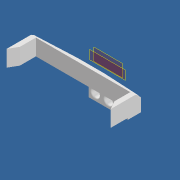
# Autodesk Inventor part: Hand
Saved by Autodesk Inventor 2020 (Build 240168000, 168)
## iProperties
Created: 2019-12-15
Part Number: Hand
Material: Generic
Document SubType Name: Modeling
Designer: Jack
Density: 1 g/cm^3
Appearance: Default
Author: Jack
Autodesk Inventor part; units mm, degrees
ref_plane "YZ Plane" through (0, 0, 0) normal (1, 0, 0) x (0, 1, 0)
ref_plane "XZ Plane" through (0, 0, 0) normal (0, 1, 0) x (-1, 0, 0)
ref_plane "XY Plane" through (0, 0, 0) normal (0, 0, 1) x (1, 0, 0)
sketch "Sketch1" plane through (0, 0, 0) normal (0, 0, 1) x (1, 0, 0)
  line L0 (32, -5) -> (-32, -5)
  line L1 (-32, -5) -> (-32, 5)
  line L2 (-32, 5) -> (32, 5)
  line L3 (32, 5) -> (32, -5)
  line L4 (32, -5) -> (-32, 5) construction
  line L5 (-32, -5) -> (32, 5) construction
  point P0 (0, 0)
  dimension "d1" = 64
  dimension "d2" = 10
  constraints: 12 end point, 2 midpoint, 2 parallel, 1 horizontal, 1 perpendicular
  measures "d1" distance of L1.end L2.end
  measures "d2" distance of L0.end L1.end
extrude "Extrusion1" add sketch "Sketch1" against normal blind 5
chamfer "Chamfer1" distance 24 distance2 3 1 edges at (32, 0, -5) measured on face at (31.5, 0, -5)
chamfer "Chamfer2" distance 24 distance2 3 1 edges at (-32, 0, -5) measured on face at (-31.5, 0, -5)
chamfer "Chamfer3" distance 3 distance2 5 1 edges at (0, 5, -5) measured on face at (0, 4.5, -5)
sketch "Sketch2" plane through (0, 0, 0) normal (0, 0, 1) x (1, 0, 0)
  line L0 (-32, 5) -> (-29, 5)
  line L1 (-29, 5) -> (-29, -5)
  line L2 (-29, -5) -> (-32, -5)
  line L3 (-32, -5) -> (-32, 5)
  line L4 (32, 5) -> (-32, 5) projected
  line L5 (-32, 5) -> (-32, -5) projected
  point P0 (0, 0)
  dimension "d14" = 3
  dimension "d15" = 10
  constraints: 8 end point, 2 collinear, 2 parallel, 1 horizontal, 1 perpendicular
  measures "d14" distance of L1.end L2.end
  measures "d15" distance of L0.end L1.end
extrude "Extrusion2" add sketch "Sketch2" along normal blind 15
chamfer "Chamfer4" distance 3 angle 60 1 edges at (-29, 0, 15) measured on face at (-29.5, 0, 15)
ref_plane "Work Plane1" through (0, 0, -15) normal (0, 0, -1) x (-1, 0, 0)
mirror "Mirror3" about plane through (0, 0, 0) normal (1, 0, 0)
ref_plane "Work Plane8" through (0, 0, -15.5) normal (0, 0, -1) x (-1, 0, 0)
sketch "Sketch19" plane through (0, 0, -15.5) normal (0, 0, -1) x (-1, 0, 0)
  line L0 (-12, -26) -> (12, -26)
  line L1 (12, -26) -> (12, -18)
  line L2 (12, -18) -> (-12, -18)
  line L3 (-12, -18) -> (-12, -26)
  line L4 (-12, -26) -> (12, -18) construction
  line L5 (12, -26) -> (-12, -18) construction
  line L6 (0, -32.2) -> (0, 11.2) projected
  line L7 (8, -5) -> (32, -5) projected
  point P0 (0, 0)
  point P1 (0, -22)
  point P2 (0, -22)
  dimension "d95" = 24
  dimension "d96" = 8
  dimension "d97" = 13
  constraints: 12 end point, 3 midpoint, 2 parallel, 1 horizontal, 1 perpendicular, 1 point on line
  measures "d95" distance of L2.end L1.end
  measures "d96" distance of L1.end L0.end
  measures "d97" distance between parallel lines of L7 L2
extrude "Extrusion9" add sketch "Sketch19" along normal blind 8
sketch "Sketch20" plane through (0, 0, -23.5) normal (0, 0, -1) x (-1, 0, 0)
  circle A0 centre (-8, -22) radius 2.4
  circle A1 centre (0, -22) radius 2.4
  circle A2 centre (8, -22) radius 2.4
  line L0 (0, -32.2) -> (0, 11.2) projected
  line L1 (12, -18) -> (-12, -18) projected
  point P0 (0, 0)
  dimension "d100" = 4.8
  dimension "d101" = 4.8
  dimension "d102" = 4.8
  dimension "d103" = 8
  dimension "d104" = 8
  dimension "d105" = 4
  constraints: 3 centre point, 2 horizontal alignment, 1 point on line
  measures "d100" diameter of A0
  measures "d101" diameter of A1
  measures "d102" diameter of A2
  measures "d103" distance of A1.centre A0.centre
  measures "d104" distance of A2.centre A1.centre
  measures "d105" distance from line of L1 A1.centre
extrude "Extrusion10" cut sketch "Sketch20" against normal blind 8
fillet "Fillet2" radius 0.7 6 edges at (10.4, -22, -23.5) (2.4, -22, -23.5) (-5.6, -22, -23.5) (2.4, -22, -15.5) (10.4, -22, -15.5) (-5.6, -22, -15.5)
loft "Loft7" add section 1 edges at (0, 2.0001, -5) (8, -1.4999, -5) (0, -5, -5) (-8, -1.5, -5) section 2 edges at (0, -18, -15.5) (12, -18, -19.5) (0, -18, -23.5) (-12, -18, -19.5)
body "Solid1"
